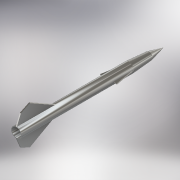
# Autodesk Inventor part: missle
Saved by Autodesk Inventor 2019 (Build 230136000, 136)
## iProperties
Created: 2020-10-17
Part Number: missle
Material: Generic
Document SubType Name: Modeling
Designer: Manoj
Density: 1 g/cm^3
Appearance: Chrome - Polished
Author: Manoj
Autodesk Inventor part; units mm, degrees
ref_plane "YZ Plane" through (0, 0, 0) normal (1, 0, 0) x (0, 1, 0)
sketch "Sketch1" plane through (0, 0, 0) normal (0, 0, 1) x (1, 0, 0)
  circle A0 centre (0, 0) radius 500
  dimension "d0" = 1000
  constraints: 1 centre point, 1 coincident
  measures "d0" diameter of A0
ref_plane "Work Plane1" through (0, 0, -2000) normal (0, 0, 1) x (1, 0, 0)
sketch "Sketch2" plane through (0, 0, -2000) normal (0, 0, 1) x (1, 0, 0)
  circle A0 centre (0, 0) radius 350
  dimension "d2" = 700
  constraints: 1 centre point, 1 coincident
  measures "d2" diameter of A0
extrude "Extrusion1" add sketch "Sketch1" along normal blind 3000
loft "Loft1" add profiles "Sketch2" section 1 edges at (-500, 0, 0)
fillet "Fillet1" radius 200 1 edges at (-500, 0, 0)
ref_plane "Work Plane2" through (0, 0, -3400) normal (0, 0, -1) x (-1, 0, 0)
sketch "Sketch3" plane through (0, 0, -3400) normal (0, 0, -1) x (-1, 0, 0)
  point P0 (0, 0)
  point P1 (0, 0)
  constraints: 1 coincident
loft "Loft2" add section 1 edges at (-350, 0, -2000) section 2 point at (0, 0, -3400)
fillet "Fillet2" radius 200 1 edges at (-350, 0, -2000)
extrude "Extrusion2" add sketch "Sketch1" along normal blind 11000
shell "Shell1" thickness 50 removed faces 1 at (-105.6691, 12.3701, 11000)
sketch "Sketch4" plane through (0, 0, 0) normal (1, 0, 0) x (0, 1, 0)
  line L0 (500, 11000) -> (-500, 11000) projected
  line L1 (-500, 11000) -> (-1448.7354, 10606.724)
  line L2 (-1448.7354, 10606.724) -> (-1894.1742, 9672.7393)
  line L3 (-1894.1742, 9672.7393) -> (-500, 7172.5343)
  line L4 (-500, 0) -> (-500, 11000) projected
  line L5 (-500, 7172.5343) -> (-500, 11000)
  line L6 (500, 11000) -> (1448.7354, 10606.724)
  line L7 (1448.7354, 10606.724) -> (1894.1742, 9672.7393)
  line L8 (1894.1742, 9672.7393) -> (500, 7172.5343)
  line L9 (500, 11000) -> (500, 7172.5343)
  line L10 (500, 0) -> (500, 11000) projected
  point P0 (0, 0)
  constraints: 16 end point, 2 collinear, 1 point on line
extrude "Extrusion3" add sketch "Sketch4" along normal mid plane 100
chamfer "Chamfer1" distance 50 angle 45 2 edges at (-50, 1197.0871, 8422.6368) (50, 1197.0871, 8422.6368)
chamfer "Chamfer2" distance 50 angle 45 2 edges at (50, -1197.0871, 8422.6368) (-50, -1197.0871, 8422.6368)
sketch "Sketch5" plane through (0, 0, 0) normal (0, 1, 0) x (-1, 0, 0)
  line L0 (-500, 0) -> (500, 0) projected
  line L1 (500, 0) -> (847.2964, 1969.6155)
  line L2 (500, 0) -> (2500, 0) construction
  line L3 (847.2964, 1969.6155) -> (500, 1969.6155)
  line L4 (500, 0) -> (500, 11000) projected
  line L5 (500, 0) -> (500, 1969.6155)
  line L6 (450, 50) -> (450, 11000) projected
  line L7 (0, -4841.3947) -> (0, -4440.4858)
  line L8 (-500, 0) -> (-847.2964, 1969.6155)
  line L9 (-847.2964, 1969.6155) -> (-500, 1969.6155)
  line L10 (-500, 0) -> (-500, 1969.6155)
  line L11 (-450, 50) -> (-450, 11000) projected
  point P0 (0, 0)
  dimension "d27" = 2000
  dimension "d28" = 80
  constraints: 16 end point, 3 symmetric about line, 2 horizontal, 2 parallel, 1 equal length, 1 point on line, 1 vertical
  measures "d27" distance of L0.end L1.end
  measures "d28" angle of L2 L1
extrude "Extrusion4" add sketch "Sketch5" along normal mid plane 100
chamfer "Chamfer3" distance 50 angle 45 4 edges at (-673.6482, -50, 984.8078) (-673.6482, 50, 984.8078) (673.6482, -50, 984.8078) (673.6482, 50, 984.8078)
body "Solid1"
